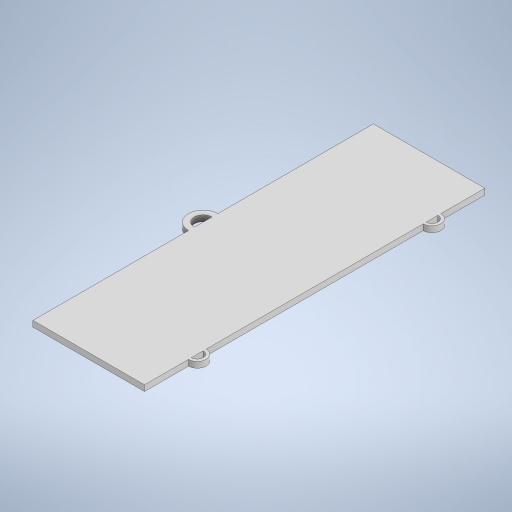
# Autodesk Inventor part: Shelf
Saved by Autodesk Inventor 2024 (Build 280153000, 153)
## iProperties
Created: 2025-02-03
Part Number: Shelf
Material: Generic
Document SubType Name: Modeling
Designer: matsk
Density: 1 g/cm^3
Appearance: Default
Author: matsk
Autodesk Inventor part; units mm, degrees
ref_plane "YZ Plane" through (0, 0, 0) normal (1, 0, 0) x (0, 1, 0)
ref_plane "XZ Plane" through (0, 0, 0) normal (0, 1, 0) x (-1, 0, 0)
ref_plane "XY Plane" through (0, 0, 0) normal (0, 0, 1) x (1, 0, 0)
sketch "Sketch1" plane through (0, 0, 0) normal (0, 1, 0) x (-1, 0, 0)
  line L0 (0, 0) -> (-9.5, 0)
  line L1 (-9.5, 0) -> (-9.5, -29)
  line L2 (-9.5, -29) -> (0, -29)
  line L3 (0, -29) -> (0, 0)
  dimension "d0" = 9.5
  dimension "d1" = 29
  constraints: 8 end point, 2 parallel, 1 horizontal, 1 perpendicular
  measures "d0" distance of L2.end L1.end
  measures "d1" distance of L1.end L0.end
extrude "Extrusion1" add sketch "Sketch1" along normal blind 0.5
sketch "Sketch3" plane through (0, 0.5, 0) normal (0, 1, 0) x (1, 0, 0)
  circle A0 centre (9.5, 24.5) radius 0.75
  circle A1 centre (9.5, 24.5) radius 0.5
  circle A2 centre (9.5, 4.5) radius 0.75
  circle A3 centre (9.5, 4.5) radius 0.5
  point P0 (0, 0)
  point P1 (9.5, 0)
  point P2 (9.5, 29)
  dimension "d6" = 1.5
  dimension "d7" = 1
  dimension "d8" = 1.5
  dimension "d9" = 1
  constraints: 4 centre point, 2 coincident
  measures "d6" diameter of A0
  measures "d7" diameter of A1
  measures "d8" diameter of A2
  measures "d9" diameter of A3
extrude "Extrusion2" add sketch "Sketch3" against normal blind 0.5
sketch "Sketch4" plane through (0, 0.5, 0) normal (0, 1, 0) x (1, 0, 0)
  line L0 (0, 29) -> (0, 0) projected
  line L1 (0, 29) -> (0, 14.5)
  circle A0 centre (0, 14.5) radius 1.25
  circle A1 centre (0, 14.5) radius 0.75
  point P0 (0, 13.75)
  point P1 (0, 15.25)
  point P2 (0, 15.75)
  point P3 (0, 13.25)
  dimension "d12" = 14.5
  dimension "d13" = 2.5
  dimension "d14" = 1.5
  constraints: 2 centre point, 2 coincident, 2 end point, 1 midpoint
  measures "d12" distance of L0.start L1.end
  measures "d13" diameter of A0
  measures "d14" diameter of A1
extrude "Extrusion3" add sketch "Sketch4" against normal blind 0.5 contours L0 A1 A0 picked at (-1.0514, 14.2719)
body "Solid1"
